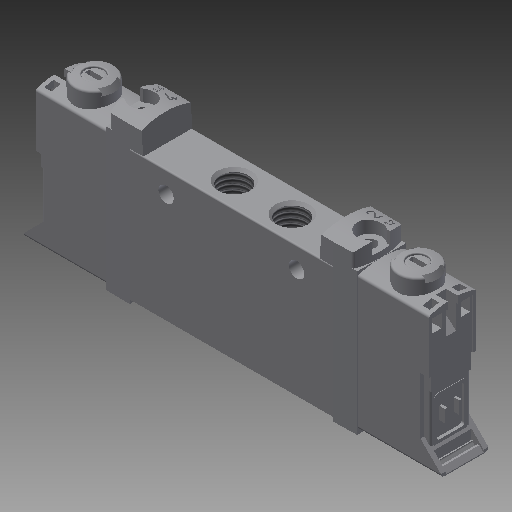
# Autodesk Inventor part: 564212 VUVG-L-10-B52---T-M7--1P3--------(G)
Saved by Autodesk Inventor 2018.3 (Build 223284000, 284)
## iProperties
Category: PARTsolutions
Company: FESTO
Created: 2019-03-04
Part Number: 564212 VUVG-L-10-B52---T-M7--1P3--------(G)
Material: Generic
Catalog Web Link: www.cadenas.de
Description: VUVG-(G)-Directional control valves for standard applications
Vendor: FESTO
Document SubType Name: Modeling
Designer: psadmin
Manufacturer: FESTO
Mass: 21.2534 g
Surface Area: 93.0719 cm^2
Volume: 21.2534 cm^3
Density: 1 g/cm^3
Appearance: PSOLRGB-192-192-192
PSOL_IDENT_0: {$CADENAS_DATA\23d-libs\festo\parts\v\vuvg\parts\vuvg_gehause.prj},277 {VTYP=3D},{NB=564212 VUVG-L-1
PSOL_IDENT_1: 0-B52---T-M7--1P3--------(G)},{LINA=564212 VUVG-L-10-B52---T-M7--1P3--------(G)},{NN=VUVG-(G)},{DATE=
PSOL_IDENT_2: 22.01.2019 12:42:35},{GEOMDATE=22.01.2019 12:42:31},{VERSION=},{LINEID=10},{WBVAR=VA,KP,BG,VF,RS,SZ,
PSOL_IDENT_3: HHB,PA,EL,NS,EA,SBS,ANZ,EZV,ZUL},{WBNUMERIC=}  {NB=564212 VUVG-L-10-B52---T-M7--1P3--------(G)},{LIN
PSOL_IDENT_4: A=564212 VUVG-L-10-B52---T-M7--1P3--------(G)},{KT=DUMMY},{TNR=564212},{TYP=VUVG},{VA=L},{KP=-},{BG=
PSOL_IDENT_5: 10},{VF=B52},{RS=-},{SZ=-},{HHB=T},{PA=M7},{EL=-},{NS=1},{EA=P3},{SBS=-},{ANZ=-},{EZV=-},{ZUL=-},{KZ
PSOL_IDENT_6: U=-},{L=42},{L1=7.5},{THREAD=7},{VERS=1},{ASP=2},{CODE=},{SCALE=0.5},{ZUL1=},{KZU1=},{ZULT='-'}
NN: VUVG-(G)
NT: Directional control valves for standard applications
NB: 564212 VUVG-L-10-B52---T-M7--1P3--------(G)
NBSYN: $TNR. $TYP.-$VA.$KP.$BG.-$VF.-$RS.$SZ.$HHB.-$PA.$EL.-$NS.$EA.-$SBS.$ANZ.-$EZV.$ZUL1.$KZU1.---(G)
LINA: 564212 VUVG-L-10-B52---T-M7--1P3--------(G)
TNR: 564212
TYP: VUVG
VA: L
KP: -
BG: 10
VF: B52
RS: -
SZ: -
HHB: T
PA: M7
EL: -
NS: 1
EA: P3
SBS: -
ANZ: -
EZV: -
ZUL: -
SUPPLIER: FESTO
ARTICLENO: 564212 VUVG-L-10-B52---T-M7--1P3--------(G)
BOMINFO: 564212 VUVG-L-10-B52---T-M7--1P3--------(G)
CREATOR: CADENAS GmbH
Title: 564212 VUVG-L-10-B52---T-M7--1P3--------(G)
Author: Cadenas PARTsolutions
Comments: Directional control valves for standard applications
Autodesk Inventor part; units mm, degrees
sketch "Sketch_53" plane through (0, 0, 0) normal (1, 0, 0) x (0, 1, 0)
  line L0 (26.7, 5.1) -> (0, 5.1)
  line L1 (0, 5.1) -> (0, -5.1)
  line L2 (0, -5.1) -> (26.7, -5.1)
  arc A0 (26.7, -5.1) -> (27, -4.8) centre (26.7, -4.8) ccw
  line L3 (27, -4.8) -> (27, 4.8)
  arc A1 (27, 4.8) -> (26.7, 5.1) centre (26.7, 4.8) ccw
  constraints: 8 end point, 4 point on circle, 2 centre point
extrude "Extrusion1" add sketch "Sketch_53" along normal mid plane 42
sketch "Sketch_54" plane through (0, 0, 0) normal (0, 0, 1) x (1, 0, 0)
  circle A0 centre (13.5, 22.6) radius 1.6
  constraints: 1 centre point
extrude "Extrusion2" cut sketch "Sketch_54" along normal mid plane 12
sketch "Sketch_55" plane through (0, 0, 0) normal (0, 0, 1) x (1, 0, 0)
  circle A0 centre (-13.5, 22.6) radius 1.6
  constraints: 1 centre point
extrude "Extrusion3" cut sketch "Sketch_55" along normal mid plane 12
sketch "Sketch_5" plane through (0, 0, 0) normal (0, 0, 1) x (1, 0, 0)
  line L0 (12.5, 0) -> (12.5, 13.5)
  line L1 (12.5, 13.5) -> (14.6, 13.5)
  line L2 (14.6, 13.5) -> (14.6, 6.8)
  line L3 (14.6, 6.8) -> (15.4585, 6.8)
  line L4 (15.4585, 6.8) -> (15.4585, 0.5415)
  line L5 (15.4585, 0.5415) -> (16, 0)
  line L6 (16, 0) -> (12.5, 0)
  line L7 (12.5, 0) -> (12.5, 13.5)
  constraints: 16 end point
sketch "Sketch_6" plane through (0, 0, 0) normal (0, 0, 1) x (1, 0, 0)
  line L0 (1.5, 0) -> (1.5, 20.0124)
  line L1 (1.5, 20.0124) -> (3.6, 18.8)
  line L2 (3.6, 18.8) -> (3.6, 6.8)
  line L3 (3.6, 6.8) -> (4.4585, 6.8)
  line L4 (4.4585, 6.8) -> (4.4585, 0.5415)
  line L5 (4.4585, 0.5415) -> (5, 0)
  line L6 (5, 0) -> (1.5, 0)
  line L7 (1.5, 0) -> (1.5, 20.0124)
  constraints: 16 end point
sketch "Sketch_7" plane through (0, 0, 0) normal (0, 0, 1) x (1, 0, 0)
  line L0 (-9.5, 0) -> (-9.5, 13.5)
  line L1 (-9.5, 13.5) -> (-7.4, 13.5)
  line L2 (-7.4, 13.5) -> (-7.4, 6.8)
  line L3 (-7.4, 6.8) -> (-6.5415, 6.8)
  line L4 (-6.5415, 6.8) -> (-6.5415, 0.5415)
  line L5 (-6.5415, 0.5415) -> (-6, 0)
  line L6 (-6, 0) -> (-9.5, 0)
  line L7 (-9.5, 0) -> (-9.5, 13.5)
  constraints: 16 end point
revolve "Revolution1" cut sketch "Sketch_5" angle 360 about axis through (12.5, 0, 0) along (0, -1, 0)
thread "Thread1" size "M7x1" class "6H" standard "ISO Metric profile" length 5.4585
revolve "Revolution2" cut sketch "Sketch_6" angle 360 about axis through (1.5, 0, 0) along (0, -1, 0)
thread "Thread2" size "M7x1" class "6H" standard "ISO Metric profile" length 5.4585
revolve "Revolution3" cut sketch "Sketch_7" angle 360 about axis through (-9.5, 0, 0) along (0, -1, 0)
thread "Thread3" size "M7x1" class "6H" standard "ISO Metric profile" length 5.4585
sketch "Sketch7" plane through (-21, 27, 4.8) normal (0, 1, 0) x (1, 0, 0)
  point P0 (16.5, 4.8)
hole "Hole1" at (-4.5, 27, 0) direction (0, -1, 0) diameter 5.9175 depth 6.8 countersink diameter 7 countersink angle 90 thread size "M7x1" class "6H" standard "ISO Metric profile"
sketch "Sketch8" plane through (-21, 27, 4.8) normal (0, 1, 0) x (1, 0, 0)
  point P0 (28.5, 4.8)
hole "Hole2" at (7.5, 27, 0) direction (0, -1, 0) diameter 5.9175 depth 6.8 countersink diameter 7 countersink angle 90 thread size "M7x1" class "6H" standard "ISO Metric profile"
sketch "Sketch9" plane through (-4.5, 20.2, 0) normal (0, 1, 0) x (1, 0, 0)
  point P0 (0, -1)
hole "Hole3" at (-4.5, 20.2, 1) direction (0, -1, 0) diameter 3 depth 6.7
sketch "Sketch10" plane through (7.5, 20.2, 0) normal (0, 1, 0) x (1, 0, 0)
  point P0 (0, 1)
hole "Hole4" at (7.5, 20.2, -1) direction (0, -1, 0) diameter 3 depth 6.7
sketch "Sketch_17" plane through (0, -0.8, 0) normal (0, 1, 0) x (1, 0, 0)
  line L0 (21, 5.125) -> (21, -5.125)
  line L1 (21, -5.125) -> (25.96, -5.0384)
  line L2 (25.96, -5.0384) -> (25.96, 5.0384)
  line L3 (25.96, 5.0384) -> (21, 5.125)
  constraints: 8 end point
extrude "Extrusion4" add sketch "Sketch_17" along normal blind 33.1
sketch "Sketch_20" plane through (0, 27, 0) normal (0, 1, 0) x (1, 0, 0)
  line L0 (18.21, 5.0763) -> (18.21, -5.0763)
  line L1 (18.21, -5.0763) -> (21, -5.125)
  line L2 (21, -5.125) -> (21, 5.125)
  line L3 (21, 5.125) -> (18.21, 5.0763)
  constraints: 8 end point
extrude "Extrusion5" add sketch "Sketch_20" along normal blind 5.7
sketch "Sketch_19" plane through (0, 0, 0) normal (1, 0, 0) x (0, 1, 0)
  arc A0 (31.3973, -5.125) -> (31.3973, 5.125) centre (17.3, 0) ccw
  line L0 (31.3973, -5.125) -> (37, -5.125)
  line L1 (37, -5.125) -> (37, 5.125)
  line L2 (37, 5.125) -> (31.3973, 5.125)
  constraints: 6 end point, 2 point on circle, 1 centre point
sketch "Sketch_30" plane through (0, 28.5, 0) normal (0, 1, 0) x (1, 0, 0)
  line L0 (21, -6.125) -> (31, -6.125)
  line L1 (31, -6.125) -> (31, 6.125)
  line L2 (31, 6.125) -> (21, 6.125)
  line L3 (21, 6.125) -> (21, 5.125)
  line L4 (21, 5.125) -> (24.7331, 5.0598)
  arc A0 (25.199, 4.7172) -> (24.7331, 5.0598) centre (24.7243, 4.5599) ccw
  arc A1 (25.199, -4.7172) -> (25.199, 4.7172) centre (10.96, 0) ccw
  arc A2 (24.7331, -5.0598) -> (25.199, -4.7172) centre (24.7243, -4.5599) ccw
  line L5 (24.7331, -5.0598) -> (21, -5.125)
  line L6 (21, -5.125) -> (21, -6.125)
  constraints: 14 end point, 6 point on circle, 3 centre point
extrude "Extrusion6" cut sketch "Sketch_30" along normal blind 5
sketch "Sketch_22" plane through (0, 0, 0) normal (0, 0, 1) x (1, 0, 0)
  line L0 (13.21, 33) -> (13.21, 27)
  line L1 (13.21, 27) -> (18.21, 27)
  line L2 (18.21, 27) -> (18.7349, 33)
  line L3 (18.7349, 33) -> (13.21, 33)
  constraints: 8 end point
extrude "Extrusion7" cut sketch "Sketch_22" along normal mid plane 12
sketch "Sketch_23" plane through (25.96, 0, 0) normal (1, 0, 0) x (0, 0, -1)
  arc A0 (-4.9, 0.7) -> (-4.2, 0) centre (-4.2, 0.7) ccw
  line L0 (-4.2, 0) -> (4.2, 0)
  arc A1 (4.2, 0) -> (4.9, 0.7) centre (4.2, 0.7) ccw
  line L1 (4.9, 0.7) -> (4.9, 27.3163)
  arc A2 (4.9, 27.3163) -> (4.5517, 27.7927) centre (4.4, 27.3163) ccw
  arc A3 (4.5517, 27.7927) -> (-4.5517, 27.7927) centre (0, 13.5) ccw
  arc A4 (-4.5517, 27.7927) -> (-4.9, 27.3163) centre (-4.4, 27.3163) ccw
  line L2 (-4.9, 27.3163) -> (-4.9, 0.7)
  constraints: 10 point on circle, 6 end point, 5 centre point
extrude "Extrusion8" add sketch "Sketch_23" along normal blind 17.2
sketch "Sketch_24" plane through (0, 0, 0) normal (0, 0, 1) x (1, 0, 0)
  line L0 (38.9067, 4.9533) -> (43.16, 0.7)
  line L1 (43.16, 0.7) -> (43.16, 30)
  line L2 (43.16, 30) -> (40.66, 30)
  line L3 (40.66, 30) -> (40.66, 16.7)
  line L4 (40.66, 16.7) -> (38.9067, 16.7)
  line L5 (38.9067, 16.7) -> (38.9067, 4.9533)
  constraints: 12 end point
extrude "Extrusion9" cut sketch "Sketch_24" along normal mid plane 12
sketch "Sketch_25" plane through (0, 13.6, 0) normal (0, 1, 0) x (1, 0, 0)
  line L0 (38.16, 4.1) -> (38.16, -4.1)
  line L1 (38.16, -4.1) -> (39.76, -4.1)
  arc A0 (39.76, -4.1) -> (40.16, -3.7) centre (39.76, -3.7) ccw
  line L2 (40.16, -3.7) -> (40.16, 3.7)
  arc A1 (40.16, 3.7) -> (39.76, 4.1) centre (39.76, 3.7) ccw
  line L3 (39.76, 4.1) -> (38.16, 4.1)
  constraints: 8 end point, 4 point on circle, 2 centre point
extrude "Extrusion10" add sketch "Sketch_25" against normal blind 12
sketch "Sketch_26" plane through (0, 13.6, 0) normal (0, 1, 0) x (1, 0, 0)
  line L0 (37.66, 4.1) -> (37.66, -4.1)
  line L1 (37.66, -4.1) -> (40.26, -4.1)
  arc A0 (40.26, -4.1) -> (40.66, -3.7) centre (40.26, -3.7) ccw
  line L2 (40.66, -3.7) -> (40.66, 3.7)
  arc A1 (40.66, 3.7) -> (40.26, 4.1) centre (40.26, 3.7) ccw
  line L3 (40.26, 4.1) -> (37.66, 4.1)
  constraints: 8 end point, 4 point on circle, 2 centre point
extrude "Extrusion11" add sketch "Sketch_26" along normal blind 3.1
sketch "Sketch_27" plane through (40.16, 0, 0) normal (1, 0, 0) x (0, 0, -1)
  line L0 (-3.45, 11.8) -> (-3.45, 0)
  line L1 (-3.45, 0) -> (3.45, 0)
  line L2 (3.45, 0) -> (3.45, 11.8)
  arc A0 (3.45, 11.8) -> (2.65, 12.6) centre (2.65, 11.8) ccw
  line L3 (2.65, 12.6) -> (-2.65, 12.6)
  arc A1 (-2.65, 12.6) -> (-3.45, 11.8) centre (-2.65, 11.8) ccw
  constraints: 8 end point, 4 point on circle, 2 centre point
extrude "Extrusion12" add sketch "Sketch_27" along normal blind 0.1
sketch "Sketch_28" plane through (40.16, 0, 0) normal (1, 0, 0) x (0, 0, -1)
  arc A0 (-2.85, 4.7) -> (-2.35, 4.2) centre (-2.35, 4.7) ccw
  line L0 (-2.35, 4.2) -> (2.35, 4.2)
  arc A1 (2.35, 4.2) -> (2.85, 4.7) centre (2.35, 4.7) ccw
  line L1 (2.85, 4.7) -> (2.85, 11.5)
  arc A2 (2.85, 11.5) -> (2.35, 12) centre (2.35, 11.5) ccw
  line L2 (2.35, 12) -> (-2.35, 12)
  arc A3 (-2.35, 12) -> (-2.85, 11.5) centre (-2.35, 11.5) ccw
  line L3 (-2.85, 11.5) -> (-2.85, 4.7)
  constraints: 8 end point, 8 point on circle, 4 centre point
extrude "Extrusion13" cut sketch "Sketch_28" along normal mid plane 1
sketch "Sketch_29" plane through (0, 9.65, 0) normal (0, 1, 0) x (1, 0, 0)
  line L0 (35.81, -1.75) -> (40.81, -1.75)
  line L1 (40.81, -1.75) -> (40.81, -1.25)
  line L2 (40.81, -1.25) -> (36.31, -1.25)
  line L3 (36.31, -1.25) -> (36.31, 1.25)
  line L4 (36.31, 1.25) -> (40.81, 1.25)
  line L5 (40.81, 1.25) -> (40.81, 1.75)
  line L6 (40.81, 1.75) -> (35.81, 1.75)
  line L7 (35.81, 1.75) -> (35.81, -1.75)
  constraints: 16 end point
extrude "Extrusion14" add sketch "Sketch_29" against normal blind 2.6
sketch "Sketch_21" plane through (0, 0, 0) normal (0, 0, 1) x (1, 0, 0)
  line L0 (23.5, -0.8) -> (23.5, 29.7)
  line L1 (23.5, 29.7) -> (24.825, 29.7)
  line L2 (24.825, 29.7) -> (24.625, -0.8)
  line L3 (24.625, -0.8) -> (23.5, -0.8)
  line L4 (23.5, -0.8) -> (23.5, 29.7)
  constraints: 10 end point
revolve "Revolution4" cut sketch "Sketch_21" angle 360 about axis through (23.5, -0.8, 0) along (0, -1, 0)
sketch "Sketch_31" plane through (0, 29.7, 0) normal (0, 1, 0) x (1, 0, 0)
  arc A0 (25.2283, 1.875) -> (25.2283, -1.875) centre (23.5, 0) ccw
  line L0 (25.2283, -1.875) -> (28.5, -1.875)
  line L1 (28.5, -1.875) -> (28.5, 1.875)
  line L2 (28.5, 1.875) -> (25.2283, 1.875)
  constraints: 6 end point, 2 point on circle, 1 centre point
extrude "Extrusion15" cut sketch "Sketch_31" along normal blind 4
sketch "Sketch_32" plane through (0, -0.8, 0) normal (0, 1, 0) x (1, 0, 0)
  line L0 (-25.96, -5.0384) -> (-21, -5.125)
  line L1 (-21, -5.125) -> (-21, 5.125)
  line L2 (-21, 5.125) -> (-25.96, 5.0384)
  line L3 (-25.96, 5.0384) -> (-25.96, -5.0384)
  constraints: 8 end point
extrude "Extrusion16" add sketch "Sketch_32" along normal blind 33.1
sketch "Sketch_33" plane through (0, 27, 0) normal (0, 1, 0) x (1, 0, 0)
  line L0 (-21, -5.125) -> (-18.21, -5.0763)
  line L1 (-18.21, -5.0763) -> (-18.21, 5.0763)
  line L2 (-18.21, 5.0763) -> (-21, 5.125)
  line L3 (-21, 5.125) -> (-21, -5.125)
  constraints: 8 end point
extrude "Extrusion17" add sketch "Sketch_33" along normal blind 5.7
extrude "Extrusion18" cut sketch "Sketch_19" along normal mid plane 64
sketch "Sketch_119" plane through (0, 29.7, 0) normal (0, 1, 0) x (1, 0, 0)
  line L0 (-26.5, -1.875) -> (-25.2283, -1.875)
  arc A0 (-25.2283, -1.875) -> (-25.2283, 1.875) centre (-23.5, 0) ccw
  line L1 (-25.2283, 1.875) -> (-26.5, 1.875)
  line L2 (-26.5, 1.875) -> (-26.5, -1.875)
  constraints: 6 end point, 2 point on circle, 1 centre point
extrude "Extrusion19" cut sketch "Sketch_119" along normal blind 4
sketch "Sketch_36" plane through (0, 0, 0) normal (0, 0, 1) x (1, 0, 0)
  line L0 (-18.7349, 33) -> (-18.21, 27)
  line L1 (-18.21, 27) -> (-13.21, 27)
  line L2 (-13.21, 27) -> (-13.21, 33)
  line L3 (-13.21, 33) -> (-18.7349, 33)
  constraints: 8 end point
extrude "Extrusion20" cut sketch "Sketch_36" along normal mid plane 12
sketch "Sketch_37" plane through (0, 28.5, 0) normal (0, 1, 0) x (1, 0, 0)
  line L0 (-31, -6.125) -> (-21, -6.125)
  line L1 (-21, -6.125) -> (-21, -5.125)
  line L2 (-21, -5.125) -> (-24.7331, -5.0598)
  arc A0 (-25.199, -4.7172) -> (-24.7331, -5.0598) centre (-24.7243, -4.5599) ccw
  arc A1 (-25.199, 4.7172) -> (-25.199, -4.7172) centre (-10.96, 0) ccw
  arc A2 (-24.7331, 5.0598) -> (-25.199, 4.7172) centre (-24.7243, 4.5599) ccw
  line L3 (-24.7331, 5.0598) -> (-21, 5.125)
  line L4 (-21, 5.125) -> (-21, 6.125)
  line L5 (-21, 6.125) -> (-31, 6.125)
  line L6 (-31, 6.125) -> (-31, -6.125)
  constraints: 14 end point, 6 point on circle, 3 centre point
extrude "Extrusion21" cut sketch "Sketch_37" along normal blind 5
sketch "Sketch_38" plane through (-25.96, 0, 0) normal (1, 0, 0) x (0, 0, -1)
  arc A0 (-4.9, 0.7) -> (-4.2, 0) centre (-4.2, 0.7) ccw
  line L0 (-4.2, 0) -> (4.2, 0)
  arc A1 (4.2, 0) -> (4.9, 0.7) centre (4.2, 0.7) ccw
  line L1 (4.9, 0.7) -> (4.9, 27.3163)
  arc A2 (4.9, 27.3163) -> (4.5517, 27.7927) centre (4.4, 27.3163) ccw
  arc A3 (4.5517, 27.7927) -> (-4.5517, 27.7927) centre (0, 13.5) ccw
  arc A4 (-4.5517, 27.7927) -> (-4.9, 27.3163) centre (-4.4, 27.3163) ccw
  line L2 (-4.9, 27.3163) -> (-4.9, 0.7)
  constraints: 10 point on circle, 6 end point, 5 centre point
extrude "Extrusion22" add sketch "Sketch_38" against normal blind 17.2
sketch "Sketch_39" plane through (0, 0, 0) normal (0, 0, 1) x (1, 0, 0)
  line L0 (-43.16, 30) -> (-43.16, 0.7)
  line L1 (-43.16, 0.7) -> (-38.9067, 4.9533)
  line L2 (-38.9067, 4.9533) -> (-38.9067, 16.7)
  line L3 (-38.9067, 16.7) -> (-40.66, 16.7)
  line L4 (-40.66, 16.7) -> (-40.66, 30)
  line L5 (-40.66, 30) -> (-43.16, 30)
  constraints: 12 end point
extrude "Extrusion23" cut sketch "Sketch_39" along normal mid plane 12
sketch "Sketch_40" plane through (0, 13.6, 0) normal (0, 1, 0) x (1, 0, 0)
  line L0 (-40.16, 3.7) -> (-40.16, -3.7)
  arc A0 (-40.16, -3.7) -> (-39.76, -4.1) centre (-39.76, -3.7) ccw
  line L1 (-39.76, -4.1) -> (-38.16, -4.1)
  line L2 (-38.16, -4.1) -> (-38.16, 4.1)
  line L3 (-38.16, 4.1) -> (-39.76, 4.1)
  arc A1 (-39.76, 4.1) -> (-40.16, 3.7) centre (-39.76, 3.7) ccw
  constraints: 8 end point, 4 point on circle, 2 centre point
extrude "Extrusion24" add sketch "Sketch_40" against normal blind 12
sketch "Sketch_41" plane through (0, 13.6, 0) normal (0, 1, 0) x (1, 0, 0)
  line L0 (-40.66, 3.7) -> (-40.66, -3.7)
  arc A0 (-40.66, -3.7) -> (-40.26, -4.1) centre (-40.26, -3.7) ccw
  line L1 (-40.26, -4.1) -> (-37.66, -4.1)
  line L2 (-37.66, -4.1) -> (-37.66, 4.1)
  line L3 (-37.66, 4.1) -> (-40.26, 4.1)
  arc A1 (-40.26, 4.1) -> (-40.66, 3.7) centre (-40.26, 3.7) ccw
  constraints: 8 end point, 4 point on circle, 2 centre point
extrude "Extrusion25" add sketch "Sketch_41" along normal blind 3.1
sketch "Sketch_42" plane through (-40.16, 0, 0) normal (1, 0, 0) x (0, 0, -1)
  line L0 (-3.45, 11.8) -> (-3.45, 0)
  line L1 (-3.45, 0) -> (3.45, 0)
  line L2 (3.45, 0) -> (3.45, 11.8)
  arc A0 (3.45, 11.8) -> (2.65, 12.6) centre (2.65, 11.8) ccw
  line L3 (2.65, 12.6) -> (-2.65, 12.6)
  arc A1 (-2.65, 12.6) -> (-3.45, 11.8) centre (-2.65, 11.8) ccw
  constraints: 8 end point, 4 point on circle, 2 centre point
extrude "Extrusion26" add sketch "Sketch_42" against normal blind 0.1
sketch "Sketch_43" plane through (-40.16, 0, 0) normal (1, 0, 0) x (0, 0, -1)
  arc A0 (-2.85, 4.7) -> (-2.35, 4.2) centre (-2.35, 4.7) ccw
  line L0 (-2.35, 4.2) -> (2.35, 4.2)
  arc A1 (2.35, 4.2) -> (2.85, 4.7) centre (2.35, 4.7) ccw
  line L1 (2.85, 4.7) -> (2.85, 11.5)
  arc A2 (2.85, 11.5) -> (2.35, 12) centre (2.35, 11.5) ccw
  line L2 (2.35, 12) -> (-2.35, 12)
  arc A3 (-2.35, 12) -> (-2.85, 11.5) centre (-2.35, 11.5) ccw
  line L3 (-2.85, 11.5) -> (-2.85, 4.7)
  constraints: 8 end point, 8 point on circle, 4 centre point
extrude "Extrusion27" cut sketch "Sketch_43" along normal mid plane 1
sketch "Sketch_44" plane through (0, 9.65, 0) normal (0, 1, 0) x (1, 0, 0)
  line L0 (-40.81, -1.25) -> (-40.81, -1.75)
  line L1 (-40.81, -1.75) -> (-35.81, -1.75)
  line L2 (-35.81, -1.75) -> (-35.81, 1.75)
  line L3 (-35.81, 1.75) -> (-40.81, 1.75)
  line L4 (-40.81, 1.75) -> (-40.81, 1.25)
  line L5 (-40.81, 1.25) -> (-36.31, 1.25)
  line L6 (-36.31, 1.25) -> (-36.31, -1.25)
  line L7 (-36.31, -1.25) -> (-40.81, -1.25)
  constraints: 16 end point
extrude "Extrusion28" add sketch "Sketch_44" against normal blind 2.6
sketch "Sketch_34" plane through (0, 0, 0) normal (0, 0, 1) x (1, 0, 0)
  line L0 (-23.5, -0.8) -> (-23.5, 29.7)
  line L1 (-23.5, 29.7) -> (-22.175, 29.7)
  line L2 (-22.175, 29.7) -> (-22.375, -0.8)
  line L3 (-22.375, -0.8) -> (-23.5, -0.8)
  line L4 (-23.5, -0.8) -> (-23.5, 29.7)
  constraints: 10 end point
revolve "Revolution5" cut sketch "Sketch_34" angle 360 about axis through (-23.5, -0.8, 0) along (0, -1, 0)
sketch "Sketch_4" plane through (0, 0, 0) normal (0, 0, 1) x (1, 0, 0)
  line L0 (33.46, 26.365) -> (33.46, 31.665)
  line L1 (33.46, 31.665) -> (37.51, 31.665)
  line L2 (37.51, 31.665) -> (37.51, 26.365)
  line L3 (37.51, 26.365) -> (33.46, 26.365)
  line L4 (33.46, 26.365) -> (33.46, 31.665)
  constraints: 10 end point
revolve "Revolution6" add sketch "Sketch_4" angle 360 about axis through (33.46, 26.365, 0) along (0, -1, 0)
sketch "Sketch_61" plane through (0, 0, 0) normal (0, 0, 1) x (1, 0, 0)
  line L0 (-33.46, 26.365) -> (-33.46, 31.665)
  line L1 (-33.46, 31.665) -> (-29.41, 31.665)
  line L2 (-29.41, 31.665) -> (-29.41, 26.365)
  line L3 (-29.41, 26.365) -> (-33.46, 26.365)
  line L4 (-33.46, 26.365) -> (-33.46, 31.665)
  constraints: 10 end point
revolve "Revolution7" add sketch "Sketch_61" angle 360 about axis through (-33.46, 26.365, 0) along (0, -1, 0)
sketch "Sketch_59" plane through (0, 0, 0) normal (0, 0, 1) x (1, 0, 0)
  line L0 (33.46, 26.365) -> (33.46, 32.365)
  line L1 (33.46, 32.365) -> (38.46, 32.365)
  line L2 (38.46, 32.365) -> (38.46, 28.865)
  line L3 (38.46, 28.865) -> (37.51, 28.865)
  line L4 (37.51, 28.865) -> (37.51, 30.9614)
  arc A0 (37.51, 30.9614) -> (37.21, 31.3487) centre (37.11, 30.9614) ccw
  arc A1 (37.21, 31.3487) -> (35.6391, 31.6659) centre (33.46, 16.825) ccw
  arc A2 (35.6391, 31.6659) -> (35.41, 31.468) centre (35.61, 31.468) ccw
  line L5 (35.41, 31.468) -> (35.41, 30.295)
  line L6 (35.41, 30.295) -> (33.46, 30.295)
  line L7 (33.46, 30.295) -> (33.46, 32.365)
  constraints: 16 end point, 6 point on circle, 3 centre point
sketch "Sketch_56" plane through (0, 0, 0) normal (0, 0, 1) x (1, 0, 0)
  line L0 (33.46, 25.41) -> (33.46, 31.41)
  line L1 (33.46, 31.41) -> (35.0042, 31.41)
  line L2 (35.0042, 31.41) -> (35.36, 31.36)
  line L3 (35.36, 31.36) -> (35.36, 29.71)
  arc A0 (35.36, 29.71) -> (35.86, 29.21) centre (35.86, 29.71) ccw
  line L4 (35.86, 29.21) -> (36.01, 29.21)
  line L5 (36.01, 29.21) -> (36.01, 25.41)
  line L6 (36.01, 25.41) -> (33.46, 25.41)
  line L7 (33.46, 25.41) -> (33.46, 31.41)
  constraints: 16 end point, 2 point on circle, 1 centre point
sketch "Sketch_57" plane through (0, 30.1, 0) normal (0, 1, 0) x (1, 0, 0)
  circle A0 centre (33.46, 0) radius 6
  arc A1 (28.8774, -2) -> (38.0426, -2) centre (33.46, 0) ccw
  line L0 (38.0426, -2) -> (36.2095, -2)
  arc A2 (36.2095, -2) -> (36.2095, 2) centre (33.46, 0) ccw
  line L1 (36.2095, 2) -> (38.0426, 2)
  arc A3 (38.0426, 2) -> (28.8774, 2) centre (33.46, 0) ccw
  line L2 (28.8774, 2) -> (30.7105, 2)
  arc A4 (30.7105, 2) -> (30.7105, -2) centre (33.46, 0) ccw
  line L3 (30.7105, -2) -> (28.8774, -2)
  constraints: 8 end point, 8 point on circle, 5 centre point
extrude "Extrusion29" cut sketch "Sketch_57" along normal blind 3
sketch "Sketch_62" plane through (0, 30.1, 0) normal (0, 1, 0) x (1, 0, 0)
  circle A0 centre (-33.46, 0) radius 6
  arc A1 (-38.0426, -2) -> (-28.8774, -2) centre (-33.46, 0) ccw
  line L0 (-28.8774, -2) -> (-30.7105, -2)
  arc A2 (-30.7105, -2) -> (-30.7105, 2) centre (-33.46, 0) ccw
  line L1 (-30.7105, 2) -> (-28.8774, 2)
  arc A3 (-28.8774, 2) -> (-38.0426, 2) centre (-33.46, 0) ccw
  line L2 (-38.0426, 2) -> (-36.2095, 2)
  arc A4 (-36.2095, 2) -> (-36.2095, -2) centre (-33.46, 0) ccw
  line L3 (-36.2095, -2) -> (-38.0426, -2)
  constraints: 8 end point, 8 point on circle, 5 centre point
extrude "Extrusion30" cut sketch "Sketch_62" along normal blind 3
sketch "Sketch_58" plane through (0, 0, 0) normal (0, 0, 1) x (1, 0, 0)
  line L0 (33.46, 26.365) -> (33.46, 31.665)
  line L1 (36.86, 31.4408) -> (36.86, 26.365)
  line L2 (36.86, 26.365) -> (37.51, 26.365)
  line L3 (37.51, 26.365) -> (37.51, 29.115)
  line L4 (37.51, 29.115) -> (37.11, 29.115)
  line L5 (37.11, 29.115) -> (37.11, 30.015)
  line L6 (37.11, 30.015) -> (37.51, 30.015)
  line L7 (37.51, 30.015) -> (37.51, 30.315)
  line L8 (37.51, 30.315) -> (36.86, 31.4408)
  constraints: 18 end point
revolve "Revolution8" add sketch "Sketch_58" angle 360 about axis through (33.46, 26.365, 0) along (0, -1, 0)
sketch "Sketch_63" plane through (0, 0, 0) normal (0, 0, 1) x (1, 0, 0)
  line L0 (-33.46, 26.365) -> (-33.46, 31.665)
  line L1 (-30.06, 31.4408) -> (-30.06, 26.365)
  line L2 (-30.06, 26.365) -> (-29.41, 26.365)
  line L3 (-29.41, 26.365) -> (-29.41, 29.115)
  line L4 (-29.41, 29.115) -> (-29.81, 29.115)
  line L5 (-29.81, 29.115) -> (-29.81, 30.015)
  line L6 (-29.81, 30.015) -> (-29.41, 30.015)
  line L7 (-29.41, 30.015) -> (-29.41, 30.315)
  line L8 (-29.41, 30.315) -> (-30.06, 31.4408)
  constraints: 18 end point
revolve "Revolution9" add sketch "Sketch_63" angle 360 about axis through (-33.46, 26.365, 0) along (0, -1, 0)
revolve "Revolution10" cut sketch "Sketch_59" angle 360 about axis through (33.46, 26.365, 0) along (0, -1, 0)
sketch "Sketch_64" plane through (0, 0, 0) normal (0, 0, 1) x (1, 0, 0)
  line L0 (-33.46, 30.295) -> (-33.46, 32.365)
  line L1 (-33.46, 32.365) -> (-28.46, 32.365)
  line L2 (-28.46, 32.365) -> (-28.46, 28.865)
  line L3 (-28.46, 28.865) -> (-29.41, 28.865)
  line L4 (-29.41, 28.865) -> (-29.41, 30.9614)
  arc A0 (-29.41, 30.9614) -> (-29.71, 31.3487) centre (-29.81, 30.9614) ccw
  arc A1 (-29.71, 31.3487) -> (-31.2809, 31.6659) centre (-33.46, 16.825) ccw
  arc A2 (-31.2809, 31.6659) -> (-31.51, 31.468) centre (-31.31, 31.468) ccw
  line L5 (-31.51, 31.468) -> (-31.51, 30.295)
  line L6 (-31.51, 30.295) -> (-33.46, 30.295)
  line L7 (-33.46, 30.295) -> (-33.46, 32.365)
  constraints: 16 end point, 6 point on circle, 3 centre point
revolve "Revolution11" cut sketch "Sketch_64" angle 360 about axis through (-33.46, 30.295, 0) along (0, -1, 0)
revolve "Revolution12" add sketch "Sketch_56" angle 360 about axis through (33.46, 25.41, 0) along (0, -1, 0)
sketch "Sketch_65" plane through (0, 0, 0) normal (0, 0, 1) x (1, 0, 0)
  line L0 (-33.46, 25.41) -> (-33.46, 31.41)
  line L1 (-33.46, 31.41) -> (-31.9158, 31.41)
  line L2 (-31.9158, 31.41) -> (-31.56, 31.36)
  line L3 (-31.56, 31.36) -> (-31.56, 29.71)
  arc A0 (-31.56, 29.71) -> (-31.06, 29.21) centre (-31.06, 29.71) ccw
  line L4 (-31.06, 29.21) -> (-30.91, 29.21)
  line L5 (-30.91, 29.21) -> (-30.91, 25.41)
  line L6 (-30.91, 25.41) -> (-33.46, 25.41)
  line L7 (-33.46, 25.41) -> (-33.46, 31.41)
  constraints: 16 end point, 2 point on circle, 1 centre point
revolve "Revolution13" add sketch "Sketch_65" angle 360 about axis through (-33.46, 25.41, 0) along (0, -1, 0)
sketch "Sketch_60" plane through (0, 31.41, 0) normal (0, 1, 0) x (1, 0, 0)
  arc A0 (32.067, 0.5) -> (32.067, -0.5) centre (33.46, 0) ccw
  line L0 (32.067, -0.5) -> (34.853, -0.5)
  arc A1 (34.853, -0.5) -> (34.853, 0.5) centre (33.46, 0) ccw
  line L1 (34.853, 0.5) -> (32.067, 0.5)
  constraints: 4 end point, 4 point on circle, 2 centre point
extrude "Extrusion31" cut sketch "Sketch_60" against normal blind 2.15
sketch "Sketch_66" plane through (0, 31.41, 0) normal (0, 1, 0) x (1, 0, 0)
  arc A0 (-34.853, 0.5) -> (-34.853, -0.5) centre (-33.46, 0) ccw
  line L0 (-34.853, -0.5) -> (-32.067, -0.5)
  arc A1 (-32.067, -0.5) -> (-32.067, 0.5) centre (-33.46, 0) ccw
  line L1 (-32.067, 0.5) -> (-34.853, 0.5)
  constraints: 4 end point, 4 point on circle, 2 centre point
extrude "Extrusion32" cut sketch "Sketch_66" against normal blind 2.15
sketch "Sketch_80" plane through (0, 0, 0) normal (0, 0, 1) x (1, 0, 0)
  line L0 (40.66, 1.2) -> (42.16, 1.2)
  line L1 (42.16, 1.2) -> (43.16, 0.2)
  line L2 (43.16, 0.2) -> (43.16, 4.2)
  line L3 (43.16, 4.2) -> (40.66, 4.2)
  line L4 (40.66, 4.2) -> (40.66, 1.2)
  constraints: 10 end point
extrude "Extrusion33" cut sketch "Sketch_80" along normal mid plane 7.8
sketch "Sketch_82" plane through (0, 0, 0) normal (0, 0, 1) x (1, 0, 0)
  line L0 (-43.16, 4.2) -> (-43.16, 0.2)
  line L1 (-43.16, 0.2) -> (-42.16, 1.2)
  line L2 (-42.16, 1.2) -> (-40.66, 1.2)
  line L3 (-40.66, 1.2) -> (-40.66, 4.2)
  line L4 (-40.66, 4.2) -> (-43.16, 4.2)
  constraints: 10 end point
extrude "Extrusion34" cut sketch "Sketch_82" along normal mid plane 7.8
sketch "Sketch_84" plane through (0, 0, 0) normal (0, 0, 1) x (1, 0, 0)
  line L0 (38.256, 28.534) -> (38.256, 23.774)
  line L1 (38.256, 23.774) -> (45.756, 17.4808)
  line L2 (45.756, 17.4808) -> (45.756, 28.534)
  line L3 (45.756, 28.534) -> (38.256, 28.534)
  constraints: 8 end point
extrude "Extrusion35" cut sketch "Sketch_84" along normal mid plane 2.1
sketch "Sketch_81" plane through (0, 0, 0) normal (0, 0, 1) x (1, 0, 0)
  line L0 (-45.756, 28.534) -> (-45.756, 17.4808)
  line L1 (-45.756, 17.4808) -> (-38.256, 23.774)
  line L2 (-38.256, 23.774) -> (-38.256, 28.534)
  line L3 (-38.256, 28.534) -> (-45.756, 28.534)
  constraints: 8 end point
extrude "Extrusion36" cut sketch "Sketch_81" along normal mid plane 2.1
sketch "Sketch_87" plane through (0, 0, 0) normal (0, 0, 1) x (1, 0, 0)
  line L0 (-43.2, 4.2) -> (-43.2, 0.2)
  line L1 (-43.2, 0.2) -> (-42.2, 1.2)
  line L2 (-42.2, 1.2) -> (-40.5, 1.2)
  line L3 (-40.5, 1.2) -> (-40.5, 4.2)
  line L4 (-40.5, 4.2) -> (-43.2, 4.2)
  constraints: 10 end point
extrude "Extrusion37" cut sketch "Sketch_87" along normal mid plane 7.8
sketch "Sketch_88" plane through (0, 0, 0) normal (0, 0, 1) x (1, 0, 0)
  arc A0 (41.3798, 1.797) -> (41.0199, 0.9693) centre (41.3972, 1.2973) ccw
  line L0 (41.0199, 0.9693) -> (41.5043, 0.412)
  arc A1 (41.5043, 0.412) -> (41.7205, 0.3157) centre (41.7157, 0.5957) ccw
  line L1 (41.7205, 0.3157) -> (41.8612, 0.3181)
  arc A2 (41.8612, 0.3181) -> (41.9556, 0.4457) centre (41.8594, 0.4181) ccw
  line L2 (41.9556, 0.4457) -> (41.8153, 0.9349)
  arc A3 (41.9079, 1.0624) -> (41.8153, 0.9349) centre (41.9114, 0.9625) ccw
  line L3 (41.9079, 1.0624) -> (45.86, 1.2004)
  line L4 (45.86, 1.2004) -> (45.86, 1.9535)
  line L5 (45.86, 1.9535) -> (41.3798, 1.797)
  constraints: 12 end point, 8 point on circle, 4 centre point
extrude "Extrusion38" cut sketch "Sketch_88" along normal mid plane 7.8
sketch "Sketch_85" plane through (0, 0, 0) normal (0, 0, 1) x (1, 0, 0)
  line L0 (-45.86, 1.9535) -> (-45.86, 1.2004)
  line L1 (-45.86, 1.2004) -> (-41.9079, 1.0624)
  arc A0 (-41.8153, 0.9349) -> (-41.9079, 1.0624) centre (-41.9114, 0.9625) ccw
  line L2 (-41.8153, 0.9349) -> (-41.9556, 0.4457)
  arc A1 (-41.9556, 0.4457) -> (-41.8612, 0.3181) centre (-41.8594, 0.4181) ccw
  line L3 (-41.8612, 0.3181) -> (-41.7205, 0.3157)
  arc A2 (-41.7205, 0.3157) -> (-41.5043, 0.412) centre (-41.7157, 0.5957) ccw
  line L4 (-41.5043, 0.412) -> (-41.0199, 0.9693)
  arc A3 (-41.0199, 0.9693) -> (-41.3798, 1.797) centre (-41.3972, 1.2973) ccw
  line L5 (-41.3798, 1.797) -> (-45.86, 1.9535)
  constraints: 12 end point, 8 point on circle, 4 centre point
extrude "Extrusion39" cut sketch "Sketch_85" along normal mid plane 7.8
sketch "Sketch_86" plane through (43.16, 0, 0) normal (1, 0, 0) x (0, 0, -1)
  line L0 (-4.25, 13.012) -> (4.25, 13.012)
  line L1 (4.25, 13.012) -> (4.25, 27.012)
  line L2 (4.25, 27.012) -> (-4.25, 27.012)
  line L3 (-4.25, 27.012) -> (-4.25, 13.012)
  constraints: 8 end point
extrude "Extrusion40" cut sketch "Sketch_86" against normal blind 2.8
sketch "Sketch_94" plane through (-43.16, 0, 0) normal (1, 0, 0) x (0, 0, -1)
  line L0 (-4.25, 13.012) -> (4.25, 13.012)
  line L1 (4.25, 13.012) -> (4.25, 27.012)
  line L2 (4.25, 27.012) -> (-4.25, 27.012)
  line L3 (-4.25, 27.012) -> (-4.25, 13.012)
  constraints: 8 end point
extrude "Extrusion41" cut sketch "Sketch_94" along normal blind 2.8
sketch "Sketch_132" plane through (38.36, 0, 0) normal (1, 0, 0) x (0, 0, -1)
  line L0 (-3.9, 31) -> (-3.9, 25)
  line L1 (-3.9, 25) -> (-2, 25)
  line L2 (-2, 25) -> (-2, 30)
  line L3 (-2, 30) -> (2, 30)
  line L4 (2, 30) -> (2, 25)
  line L5 (2, 25) -> (3.9, 25)
  line L6 (3.9, 25) -> (3.9, 31)
  line L7 (3.9, 31) -> (-3.9, 31)
  constraints: 16 end point
extrude "Extrusion42" cut sketch "Sketch_132" along normal blind 1.5
sketch "Sketch_133" plane through (-38.36, 0, 0) normal (1, 0, 0) x (0, 0, -1)
  line L0 (-3.9, 31) -> (-3.9, 25)
  line L1 (-3.9, 25) -> (-2, 25)
  line L2 (-2, 25) -> (-2, 30)
  line L3 (-2, 30) -> (2, 30)
  line L4 (2, 30) -> (2, 25)
  line L5 (2, 25) -> (3.9, 25)
  line L6 (3.9, 25) -> (3.9, 31)
  line L7 (3.9, 31) -> (-3.9, 31)
  constraints: 16 end point
extrude "Extrusion43" cut sketch "Sketch_133" against normal blind 1.5
sketch "Sketch_134" plane through (38.36, 0, 0) normal (1, 0, 0) x (0, 0, -1)
  line L0 (-3.9, 27) -> (-3.9, 24)
  line L1 (-3.9, 24) -> (-2, 24)
  line L2 (-2, 24) -> (-2, 27)
  line L3 (-2, 27) -> (-3.9, 27)
  constraints: 8 end point
extrude "Extrusion44" cut sketch "Sketch_134" along normal blind 3
sketch "Sketch_135" plane through (38.36, 0, 0) normal (1, 0, 0) x (0, 0, -1)
  line L0 (2, 27) -> (2, 24)
  line L1 (2, 24) -> (3.9, 24)
  line L2 (3.9, 24) -> (3.9, 27)
  line L3 (3.9, 27) -> (2, 27)
  constraints: 8 end point
extrude "Extrusion45" cut sketch "Sketch_135" along normal blind 3
sketch "Sketch_136" plane through (-38.36, 0, 0) normal (1, 0, 0) x (0, 0, -1)
  line L0 (-3.9, 27) -> (-3.9, 24)
  line L1 (-3.9, 24) -> (-2, 24)
  line L2 (-2, 24) -> (-2, 27)
  line L3 (-2, 27) -> (-3.9, 27)
  constraints: 8 end point
extrude "Extrusion46" cut sketch "Sketch_136" against normal blind 3
sketch "Sketch_137" plane through (-38.36, 0, 0) normal (1, 0, 0) x (0, 0, -1)
  line L0 (2, 27) -> (2, 24)
  line L1 (2, 24) -> (3.9, 24)
  line L2 (3.9, 24) -> (3.9, 27)
  line L3 (3.9, 27) -> (2, 27)
  constraints: 8 end point
extrude "Extrusion47" cut sketch "Sketch_137" against normal blind 3
sketch "Sketch_12" plane through (0, 31.7, 0) normal (0, 1, 0) x (1, 0, 0)
  line L0 (-24.6, 3.175) -> (-24.138, 2.8515)
  line L1 (-24.138, 2.8515) -> (-24.0676, 2.9522)
  line L2 (-24.0676, 2.9522) -> (-24.3858, 3.175)
  line L3 (-24.3858, 3.175) -> (-23.55, 3.175)
  line L4 (-23.55, 3.175) -> (-23.55, 2.875)
  line L5 (-23.55, 2.875) -> (-23.4, 2.875)
  line L6 (-23.4, 2.875) -> (-23.4, 3.625)
  line L7 (-23.4, 3.625) -> (-23.55, 3.625)
  line L8 (-23.55, 3.625) -> (-23.55, 3.325)
  line L9 (-23.55, 3.325) -> (-24.6, 3.325)
  line L10 (-24.6, 3.325) -> (-24.6, 3.175)
  constraints: 22 end point
extrude "Extrusion48" cut sketch "Sketch_12" along normal mid plane 2
sketch "Sketch_68" plane through (0, 31.7, 0) normal (0, 1, 0) x (1, 0, 0)
  line L0 (-24.6, 4.2508) -> (-23.7083, 3.835)
  line L1 (-23.7083, 3.835) -> (-23.6, 3.835)
  line L2 (-23.6, 3.835) -> (-23.6, 4.25)
  line L3 (-23.6, 4.25) -> (-23.4, 4.25)
  line L4 (-23.4, 4.25) -> (-23.4, 4.4)
  line L5 (-23.4, 4.4) -> (-23.6, 4.4)
  line L6 (-23.6, 4.4) -> (-23.6, 4.665)
  line L7 (-23.6, 4.665) -> (-23.75, 4.665)
  line L8 (-23.75, 4.665) -> (-23.75, 4.4)
  line L9 (-23.75, 4.4) -> (-23.9, 4.4)
  line L10 (-23.9, 4.4) -> (-23.9, 4.25)
  line L11 (-23.9, 4.25) -> (-23.75, 4.25)
  line L12 (-23.75, 4.25) -> (-23.75, 4.0199)
  line L13 (-23.75, 4.0199) -> (-24.6, 4.4163)
  line L14 (-24.6, 4.4163) -> (-24.6, 4.2508)
  constraints: 30 end point
extrude "Extrusion49" cut sketch "Sketch_68" along normal mid plane 2
sketch "Sketch_101" plane through (0, 31.7, 0) normal (0, 1, 0) x (1, 0, 0)
  line L0 (-22.4, 3.5016) -> (-20.6166, 2.67)
  line L1 (-20.6166, 2.67) -> (-20.4, 2.67)
  line L2 (-20.4, 2.67) -> (-20.4, 3.5)
  line L3 (-20.4, 3.5) -> (-20, 3.5)
  line L4 (-20, 3.5) -> (-20, 3.8)
  line L5 (-20, 3.8) -> (-20.4, 3.8)
  line L6 (-20.4, 3.8) -> (-20.4, 4.33)
  line L7 (-20.4, 4.33) -> (-20.7, 4.33)
  line L8 (-20.7, 4.33) -> (-20.7, 3.8)
  line L9 (-20.7, 3.8) -> (-21, 3.8)
  line L10 (-21, 3.8) -> (-21, 3.5)
  line L11 (-21, 3.5) -> (-20.7, 3.5)
  line L12 (-20.7, 3.5) -> (-20.7, 3.0399)
  line L13 (-20.7, 3.0399) -> (-22.4, 3.8326)
  line L14 (-22.4, 3.8326) -> (-22.4, 3.5016)
  constraints: 30 end point
extrude "Extrusion50" cut sketch "Sketch_101" along normal mid plane 2
sketch "Sketch_102" plane through (0, 31.7, 0) normal (0, 1, 0) x (1, 0, 0)
  arc A0 (20.8536, 3.9962) -> (20.325, 2.775) centre (20.325, 3.5) ccw
  line L0 (20.325, 2.775) -> (20.325, 3.075)
  arc A1 (20.6349, 3.7909) -> (20.325, 3.075) centre (20.325, 3.5) ccw
  line L1 (20.6349, 3.7909) -> (21.5885, 2.775)
  line L2 (21.5885, 2.775) -> (22, 2.775)
  line L3 (22, 2.775) -> (22, 4.225)
  line L4 (22, 4.225) -> (21.7, 4.225)
  line L5 (21.7, 4.225) -> (21.7, 3.0946)
  line L6 (21.7, 3.0946) -> (20.8536, 3.9962)
  constraints: 14 end point, 4 point on circle, 2 centre point
extrude "Extrusion51" cut sketch "Sketch_102" along normal mid plane 2
sketch "Sketch_103" plane through (0, 31.7, 0) normal (0, 1, 0) x (1, 0, 0)
  line L0 (23.3, 3.175) -> (23.762, 2.8515)
  line L1 (23.762, 2.8515) -> (23.8324, 2.9522)
  line L2 (23.8324, 2.9522) -> (23.5142, 3.175)
  line L3 (23.5142, 3.175) -> (24.35, 3.175)
  line L4 (24.35, 3.175) -> (24.35, 2.875)
  line L5 (24.35, 2.875) -> (24.5, 2.875)
  line L6 (24.5, 2.875) -> (24.5, 3.625)
  line L7 (24.5, 3.625) -> (24.35, 3.625)
  line L8 (24.35, 3.625) -> (24.35, 3.325)
  line L9 (24.35, 3.325) -> (23.3, 3.325)
  line L10 (23.3, 3.325) -> (23.3, 3.175)
  constraints: 22 end point
extrude "Extrusion52" cut sketch "Sketch_103" along normal mid plane 2
sketch "Sketch_104" plane through (0, 31.7, 0) normal (0, 1, 0) x (1, 0, 0)
  arc A0 (23.9268, 4.4981) -> (23.6625, 3.8875) centre (23.6625, 4.25) ccw
  line L0 (23.6625, 3.8875) -> (23.6625, 4.0375)
  arc A1 (23.8174, 4.3954) -> (23.6625, 4.0375) centre (23.6625, 4.25) ccw
  line L1 (23.8174, 4.3954) -> (24.2943, 3.8875)
  line L2 (24.2943, 3.8875) -> (24.5, 3.8875)
  line L3 (24.5, 3.8875) -> (24.5, 4.6125)
  line L4 (24.5, 4.6125) -> (24.35, 4.6125)
  line L5 (24.35, 4.6125) -> (24.35, 4.0473)
  line L6 (24.35, 4.0473) -> (23.9268, 4.4981)
  constraints: 14 end point, 4 point on circle, 2 centre point
extrude "Extrusion53" cut sketch "Sketch_104" along normal mid plane 2
ref_plane "DICHTUNG_XY" through (1.5, 0, 0) normal (0, 1, 0) x (1, 0, 0)
ref_plane "DICHTUNG_YZ" through (1.5, 0, 0) normal (1, 0, 0) x (0, 0, -1)
ref_plane "DICHTUNG_ZX" through (1.5, 0, 0) normal (0, 0, -1) x (0, 1, 0)
ref_plane "GEHAUSE_XY" through (0, 0, 0) normal (0, 1, 0) x (1, 0, 0)
ref_plane "GEHAUSE_YZ" through (0, 0, 0) normal (1, 0, 0) x (0, 0, -1)
ref_plane "GEHAUSE_ZX" through (0, 0, 0) normal (0, 0, -1) x (0, 1, 0)
ref_plane "HHB1_XY" through (33.46, 31.66, 0) normal (0, 1, 0) x (1, 0, 0)
ref_plane "HHB1_YZ" through (33.46, 31.66, 0) normal (1, 0, 0) x (0, 0, -1)
ref_plane "HHB1_ZX" through (33.46, 31.66, 0) normal (0, 0, -1) x (0, 1, 0)
ref_plane "HHB2_XY" through (-33.46, 31.66, 0) normal (0, 1, 0) x (1, 0, 0)
ref_plane "HHB2_YZ" through (-33.46, 31.66, 0) normal (1, 0, 0) x (0, 0, -1)
ref_plane "HHB2_ZX" through (-33.46, 31.66, 0) normal (0, 0, -1) x (0, 1, 0)
ref_plane "NEBV1_XY" through (45.896, 24.712, 0) normal (1, 0, 0) x (0, 0, -1)
ref_plane "NEBV1_YZ" through (45.896, 24.712, 0) normal (0, 0, -1) x (0, 1, 0)
ref_plane "NEBV1_ZX" through (45.896, 24.712, 0) normal (0, 1, 0) x (1, 0, 0)
ref_plane "NEBV2_XY" through (-45.896, 24.712, 0) normal (-1, 0, 0) x (0, 0, -1)
ref_plane "NEBV2_YZ" through (-45.896, 24.712, 0) normal (0, 0, -1) x (0, -1, 0)
ref_plane "NEBV2_ZX" through (-45.896, 24.712, 0) normal (0, -1, 0) x (-1, 0, 0)
ref_plane "QS_K1_XY" through (1.5, 0, 0) normal (0, 1, 0) x (1, 0, 0)
ref_plane "QS_K1_YZ" through (1.5, 0, 0) normal (1, 0, 0) x (0, 0, -1)
ref_plane "QS_K1_ZX" through (1.5, 0, 0) normal (0, 0, -1) x (0, 1, 0)
ref_plane "QS_K1214_XY" through (-14.2, 27, -1.605) normal (0, -1, 0) x (1, 0, 0)
ref_plane "QS_K1214_YZ" through (-14.2, 27, -1.605) normal (1, 0, 0) x (0, 0, 1)
ref_plane "QS_K1214_ZX" through (-14.2, 27, -1.605) normal (0, 0, 1) x (0, -1, 0)
ref_plane "QS_K2_XY" through (7.5, 27, 0) normal (0, -1, 0) x (1, 0, 0)
ref_plane "QS_K2_YZ" through (7.5, 27, 0) normal (1, 0, 0) x (0, 0, 1)
ref_plane "QS_K2_ZX" through (7.5, 27, 0) normal (0, 0, 1) x (0, -1, 0)
ref_plane "QS_K3_XY" through (12.5, 0, 0) normal (0, 1, 0) x (1, 0, 0)
ref_plane "QS_K3_YZ" through (12.5, 0, 0) normal (1, 0, 0) x (0, 0, -1)
ref_plane "QS_K3_ZX" through (12.5, 0, 0) normal (0, 0, -1) x (0, 1, 0)
ref_plane "QS_K4_XY" through (-4.5, 27, 0) normal (0, -1, 0) x (1, 0, 0)
ref_plane "QS_K4_YZ" through (-4.5, 27, 0) normal (1, 0, 0) x (0, 0, 1)
ref_plane "QS_K4_ZX" through (-4.5, 27, 0) normal (0, 0, 1) x (0, -1, 0)
ref_plane "QS_K5_XY" through (-9.5, 0, 0) normal (0, 1, 0) x (1, 0, 0)
ref_plane "QS_K5_YZ" through (-9.5, 0, 0) normal (1, 0, 0) x (0, 0, -1)
ref_plane "QS_K5_ZX" through (-9.5, 0, 0) normal (0, 0, -1) x (0, 1, 0)
ref_plane "SCREW1_XY" through (23.5, 29.7, 0) normal (0, 1, 0) x (1, 0, 0)
ref_plane "SCREW1_YZ" through (23.5, 29.7, 0) normal (1, 0, 0) x (0, 0, -1)
ref_plane "SCREW1_ZX" through (23.5, 29.7, 0) normal (0, 0, -1) x (0, 1, 0)
ref_plane "SCREW2_XY" through (-23.5, 29.7, 0) normal (0, 1, 0) x (1, 0, 0)
ref_plane "SCREW2_YZ" through (-23.5, 29.7, 0) normal (1, 0, 0) x (0, 0, -1)
ref_plane "SCREW2_ZX" through (-23.5, 29.7, 0) normal (0, 0, -1) x (0, 1, 0)
ref_plane "VAVE1_XY" through (-41.58, 1.2, 0) normal (0, 1, 0) x (1, 0, 0)
ref_plane "VAVE1_YZ" through (-41.58, 1.2, 0) normal (1, 0, 0) x (0, 0, -1)
ref_plane "VAVE1_ZX" through (-41.58, 1.2, 0) normal (0, 0, -1) x (0, 1, 0)
ref_plane "VAVE2_XY" through (41.58, 1.2, 0) normal (0, 1, 0) x (1, 0, 0)
ref_plane "VAVE2_YZ" through (41.58, 1.2, 0) normal (1, 0, 0) x (0, 0, -1)
ref_plane "VAVE2_ZX" through (41.58, 1.2, 0) normal (0, 0, -1) x (0, 1, 0)
body "Solid1"
